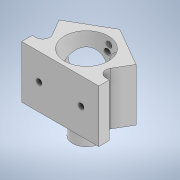
# Autodesk Inventor part: Część16
Saved by Autodesk Inventor 2021 (Build 250183000, 183)
## iProperties
Created: 2023-10-25
Part Number: Część16
Material: Ogólny
Document SubType Name: Modeling
Designer: Jakub
Density: 1 g/cm^3
Appearance: Domyślna
Author: Jakub
Autodesk Inventor part; units mm, degrees
ref_plane "YZ Plane" through (0, 0, 0) normal (1, 0, 0) x (0, 1, 0)
ref_plane "XZ Plane" through (0, 0, 0) normal (0, 1, 0) x (-1, 0, 0)
ref_plane "XY Plane" through (0, 0, 0) normal (0, 0, 1) x (1, 0, 0)
sketch "Szkic1" plane through (0, 0, 0) normal (0, 1, 0) x (-1, 0, 0)
  line L0 (0, 0) -> (-11, 0)
  line L1 (-11, 0) -> (11, 0)
  line L2 (11, 0) -> (11, -3)
  line L3 (-11, 0) -> (-11, -3)
  line L4 (-11, -3) -> (-10, -3)
  line L5 (11, -3) -> (10, -3)
  line L6 (10, -3) -> (10, -5)
  line L7 (-10, -3) -> (-10, -5)
  circle A0 centre (-10, -5) radius 2
  circle A1 centre (10, -5) radius 2
  line L8 (0, 0) -> (0, -17)
  line L9 (0, -17) -> (11, -17)
  line L10 (11, -17) -> (-11, -17)
  line L11 (0, -17) -> (11, -10.6491)
  line L12 (0, -17) -> (12.7017, -17) construction
  line L13 (0, -17) -> (-11, -10.6491)
  line L14 (-11, -10.6491) -> (-8.2757, -6.0133)
  line L15 (11, -10.6491) -> (8.2757, -6.0133)
  dimension "d8" = 4
  dimension "d9" = 4
  dimension "d0" = 11
  dimension "d1" = 22
  dimension "d2" = 3
  dimension "d3" = 3
  dimension "d4" = 1
  dimension "d5" = 1
  dimension "d6" = 2
  dimension "d7" = 2
  dimension "d10" = 17
  dimension "d11" = 22
  dimension "d12" = 30
  constraints: 32 end point, 5 horizontal, 3 vertical, 2 coincident, 2 perpendicular, 2 point on line, 1 equal length, 8 other
  measures "d0" distance of L0.start L0.end
  measures "d1" distance of L0.end L1.end
  measures "d2" distance of L1.end L2.end
  measures "d3" distance of L0.end L3.end
  measures "d4" distance of L3.end L4.end
  measures "d5" distance of L2.end L5.end
  measures "d6" distance of L5.end L6.end
  measures "d7" distance of L4.end L7.end
  measures "d10" distance of L0.start L8.end
  measures "d11" distance of L9.end L10.end
  measures "d12" angle of L12 L11
extrude "Wyciągnięcie proste1" add sketch "Szkic1" along normal blind 15 contours L8 L13 L14 A0 L4 L3 L0 | L1 L2 L5 A1 L15 L11 L8
sketch "Szkic2" plane through (0, 0, 0) normal (0, -1, 0) x (1, 0, 0)
  line L0 (0, 0) -> (0, -7.5)
  circle A0 centre (0, -7.5) radius 3.9607
  dimension "d15" = 7.5
  constraints: 2 end point, 1 centre point, 1 coincident, 1 vertical
  measures "d15" distance of L0.start L0.end
extrude "Wyciągnięcie proste2" add sketch "Szkic2" along normal blind 6.5
sketch "Szkic3" plane through (0, -6.5, -7.5) normal (0, -1, 0) x (1, 0, 0)
  circle A0 centre (0, 0) radius 3
  point P0 (0, 7.5)
  dimension "d18" = 6
  constraints: 1 centre point
  measures "d18" diameter of A0
extrude "Wyciągnięcie proste3" cut sketch "Szkic3" against normal blind 21.5
sketch "Szkic4" plane through (0, 15, 0) normal (0, 1, 0) x (1, 0, 0)
  circle A0 centre (0, 7.5) radius 6.25
  point P0 (0, 0)
  dimension "d21" = 12.5
  constraints: 1 centre point
  measures "d21" diameter of A0
fillet "Zaokrąglenie1" radius 1 1 edges at (-3.9607, 0, -7.5)
extrude "Wyciągnięcie proste4" cut sketch "Szkic4" against normal blind 14
sketch "Szkic5" plane through (0, 0, -17) normal (0.5, 0, -0.8660254) x (-0.8660254, 0, -0.5)
  line L0 (-12.7017, 15) -> (0, 15) projected
  line L1 (-6.3509, 15) -> (-6.3509, 8.5)
  circle A0 centre (-6.3509, 8.5) radius 4.5
  point P0 (-8.5, 0)
  dimension "d25" = 6.5
  dimension "d26" = 9
  constraints: 2 end point, 1 centre point, 1 coincident, 1 midpoint, 1 vertical
  measures "d25" distance of L1.start L1.end
  measures "d26" diameter of A0
extrude "Wyciągnięcie proste5" cut sketch "Szkic5" against normal blind 9.25
sketch "Szkic6" plane through (-11, 0, -10.6491) normal (-0.5, 0, -0.8660254) x (-0.8660254, 0, 0.5)
  line L0 (-14.2017, 15) -> (-1.7017, 15) projected
  line L1 (-6.35, 15) -> (-6.35, 0)
  line L2 (-12.9124, 0) -> (-2.991, 0) projected
  line L3 (-6.35, 0) -> (-2.991, 0)
  line L4 (-2.991, 0) -> (-2.991, 6.5)
  circle A0 centre (-6.35, 6.5) radius 4.5
  point P0 (-4.2017, 0)
  dimension "d6" = 2
  dimension "d29" = 6.5
  dimension "d30" = 9
  constraints: 6 end point, 2 point on line, 1 centre point, 1 collinear, 1 perpendicular, 1 vertical
  measures "d29" distance of L2.end L4.end
  measures "d30" diameter of A0
extrude "Wyciągnięcie proste6" cut sketch "Szkic6" against normal blind 9.25 contours A0 L1 | L1 A0
sketch "Szkic7" plane through (0, 0, -17) normal (0.5, 0, -0.8660254) x (-0.8660254, 0, -0.5)
  line L0 (-1.8509, 4) -> (-1.8509, 13)
  line L1 (-1.8509, 13) -> (-11, 13)
  line L2 (-11, 15) -> (-11, 1) projected
  line L3 (-1.8509, 4) -> (-11, 4)
  line L4 (-11, 4) -> (-11, 13)
  point P0 (-8.5, 0)
  constraints: 8 end point, 2 perpendicular, 1 horizontal, 1 point on line, 1 vertical
hole "Otwór1" at (1.6029, 4, -16.0746) at (1.6029, 13, -16.0746) at (9.5263, 13, -11.5) at (9.5263, 4, -11.5) direction (-0.5, 0, 0.8660254) diameter 1.567 depth 4 tip angle 90 thread size "M2x0.4" class "6H" standard "ANSI Metric M Profile"
sketch "Szkic8" plane through (-11, 0, -10.6491) normal (-0.5, 0, -0.8660254) x (-0.8660254, 0, 0.5)
  line L0 (-10.85, 11) -> (-10.85, 2)
  line L1 (-10.85, 11) -> (-1.85, 11)
  line L2 (-1.85, 11) -> (-1.85, 2)
  line L3 (-1.85, 2) -> (-10.85, 2)
  point P0 (-4.2017, 0)
  point P1 (-6.35, 2)
  dimension "d40" = 9
  dimension "d41" = 9
  constraints: 8 end point, 2 perpendicular, 1 vertical
  measures "d40" distance of L0.start L1.end
  measures "d41" distance of L1.end L2.end
hole "Otwór2" at (-9.3979, 2, -11.5741) at (-9.3979, 11, -11.5741) at (-1.6036, 11, -16.0741) at (-1.6036, 2, -16.0741) direction (0.5, 0, 0.8660254) diameter 1.567 depth 4 tip angle 90 thread size "M2x0.4" class "6H" standard "ANSI Metric M Profile"
sketch "Szkic9" plane through (-11, 0, 0) normal (0, 0, 1) x (1, 0, 0)
  line L0 (0, 0) -> (0, 15) projected
  line L1 (0, 15) -> (0, 7.5)
  line L2 (0, 15) -> (7.5, 15) construction
  line L3 (0, 7.5) -> (22, 7.5)
  line L4 (22, 0) -> (22, 15) projected
  line L5 (1, 15) -> (0, 15) projected
  line L6 (0, 15) -> (5, 15)
  line L7 (22, 15) -> (21, 15) projected
  line L8 (22, 15) -> (17, 15)
  line L9 (5, 15) -> (5, 7.5)
  line L10 (17, 15) -> (17, 7.5)
  point P0 (11, 0)
  dimension "d49" = 7.5
  dimension "d50" = 90
  dimension "d51" = 5
  dimension "d52" = 5
  constraints: 14 end point, 3 collinear, 2 point on line, 1 horizontal, 1 midpoint, 1 parallel, 1 perpendicular, 1 vertical
  measures "d49" distance of L0.end L1.end
  measures "d50" angle of L1 L2
  measures "d51" distance of L0.end L6.end
  measures "d52" distance of L4.end L8.end
hole "Otwór3" at (-6, 7.5, 0) at (6, 7.5, 0) direction (0, 0, -1) diameter 1.567 depth 4 tip angle 90 thread size "M2x0.4" class "6H" standard "ANSI Metric M Profile"
